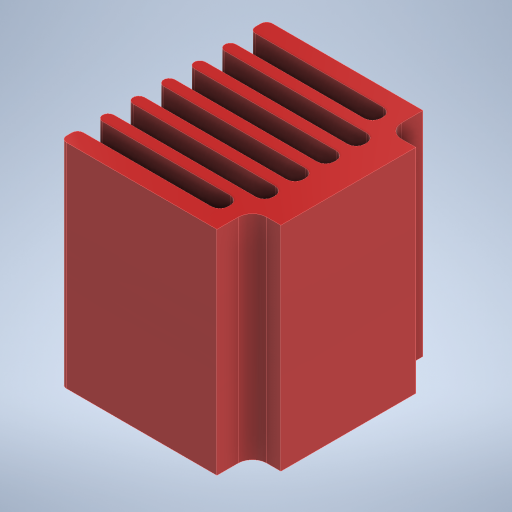
# Autodesk Inventor part: Heatsink5160Pro
Saved by Autodesk Inventor 2023.1 (Build 271208000, 208)
## iProperties
Created: 2022-09-12
Part Number: Heatsink5160Pro
Material: Generisch
Document SubType Name: Modeling
Designer: Rama
Density: 1 g/cm^3
Appearance: Rot
Author: Rama
Autodesk Inventor part; units mm, degrees
ref_plane "YZ Plane" through (0, 0, 0) normal (1, 0, 0) x (0, 1, 0)
ref_plane "XZ Plane" through (0, 0, 0) normal (0, 1, 0) x (-1, 0, 0)
ref_plane "XY Plane" through (0, 0, 0) normal (0, 0, 1) x (1, 0, 0)
sketch "Skizze1" plane through (0, 0, 0) normal (0, 1, 0) x (-1, 0, 0)
  line L0 (6.5, 7.25) -> (-6.5, 7.25)
  line L1 (-6.5, 7.25) -> (-6.5, -7.25)
  line L2 (-6.5, -7.25) -> (6.5, -7.25)
  line L3 (6.5, -7.25) -> (6.5, 7.25)
  line L4 (6.5, 7.25) -> (-6.5, -7.25) construction
  line L5 (-6.5, 7.25) -> (6.5, -7.25) construction
  line L6 (-6.5, -7.25) -> (-4.5, -7.25)
  line L7 (-4.5, -7.25) -> (-4.5, -5.75)
  line L8 (-5.5, -4.75) -> (-6.5, -4.75)
  line L9 (-6.5, -4.75) -> (-6.5, -7.25)
  arc A0 (-4.5, -5.75) -> (-5.5, -4.75) centre (-5.5, -5.75) ccw
  line L10 (-6.5, 0) -> (-5.3357, 0)
  line L11 (6.5, -4.7) -> (-2.9, -4.7)
  line L12 (-3.5, -5.3) -> (-3.5, -5.45)
  line L13 (-2.9, -6.05) -> (6.5, -6.05)
  line L14 (6.5, -6.05) -> (6.5, -4.7)
  line L15 (6.5, -2.55) -> (-3.9, -2.55)
  line L16 (-4.5, -3.15) -> (-4.5, -3.3)
  line L17 (-3.9, -3.9) -> (6.5, -3.9)
  line L18 (6.5, -3.9) -> (6.5, -2.55)
  line L19 (6.5, -0.4) -> (-3.9, -0.4)
  line L20 (-4.5, -1) -> (-4.5, -1.15)
  line L21 (-3.9, -1.75) -> (6.5, -1.75)
  line L22 (6.5, -1.75) -> (6.5, -0.4)
  line L23 (-4.5, 7.25) -> (-4.5, 5.75)
  line L24 (-5.5, 4.75) -> (-6.5, 4.75)
  arc A1 (-5.5, 4.75) -> (-4.5, 5.75) centre (-5.5, 5.75) ccw
  line L25 (6.5, 4.7) -> (-2.9, 4.7)
  line L26 (-3.5, 5.3) -> (-3.5, 5.45)
  line L27 (-2.9, 6.05) -> (6.5, 6.05)
  line L28 (6.5, 2.55) -> (-3.9, 2.55)
  line L29 (-4.5, 3.15) -> (-4.5, 3.3)
  line L30 (-3.9, 3.9) -> (6.5, 3.9)
  line L31 (6.5, 0.4) -> (-3.9, 0.4)
  line L32 (-4.5, 1) -> (-4.5, 1.15)
  line L33 (-3.9, 1.75) -> (6.5, 1.75)
  arc A2 (-2.9, 6.05) -> (-3.5, 5.45) centre (-2.9, 5.45) ccw
  arc A3 (-3.5, 5.3) -> (-2.9, 4.7) centre (-2.9, 5.3) ccw
  arc A4 (-3.9, 3.9) -> (-4.5, 3.3) centre (-3.9, 3.3) ccw
  arc A5 (-4.5, 3.15) -> (-3.9, 2.55) centre (-3.9, 3.15) ccw
  arc A6 (-3.9, 1.75) -> (-4.5, 1.15) centre (-3.9, 1.15) ccw
  arc A7 (-4.5, 1) -> (-3.9, 0.4) centre (-3.9, 1) ccw
  arc A8 (-3.9, -0.4) -> (-4.5, -1) centre (-3.9, -1) ccw
  arc A9 (-4.5, -1.15) -> (-3.9, -1.75) centre (-3.9, -1.15) ccw
  arc A10 (-3.9, -2.55) -> (-4.5, -3.15) centre (-3.9, -3.15) ccw
  arc A11 (-4.5, -3.3) -> (-3.9, -3.9) centre (-3.9, -3.3) ccw
  arc A12 (-2.9, -4.7) -> (-3.5, -5.3) centre (-2.9, -5.3) ccw
  arc A13 (-3.5, -5.45) -> (-2.9, -6.05) centre (-2.9, -5.45) ccw
  point P0 (0, 0)
  point P1 (-4.5, -4.75)
  point P2 (-3.5, -6.05)
  point P3 (-3.5, -4.7)
  point P4 (-4.5, -3.9)
  point P5 (-4.5, -2.55)
  point P6 (-4.5, -1.75)
  point P7 (-4.5, -0.4)
  point P8 (-3.5, 6.05)
  point P9 (-3.5, 4.7)
  point P10 (-4.5, 3.9)
  point P11 (-4.5, 2.55)
  point P12 (-4.5, 1.75)
  point P13 (-4.5, 0.4)
  point P14 (6.5, -3.9)
  point P15 (6.5, -1.75)
  point P16 (6.5, 1.75)
  dimension "d0" = 13
  dimension "d1" = 14.5
  dimension "d2" = 2
  dimension "d3" = 2.5
  dimension "d4" = 1
  dimension "d5" = 10
  dimension "d6" = 1.35
  dimension "d7" = 11
  dimension "d8" = 1.35
  dimension "d9" = 1.2
  dimension "d10" = 0.8
  dimension "d11" = 11
  dimension "d12" = 1.35
  dimension "d13" = 0.8
  dimension "d14" = 0.8
  dimension "d15" = 0.6
  constraints: 68 end point, 29 point on line, 28 point on circle, 26 tangent, 17 symmetric about line, 14 centre point, 11 equal radius, 10 parallel, 6 horizontal, 5 perpendicular, 3 midpoint, 1 other
  measures "d0" distance of L2.end L1.end
  measures "d1" distance of L1.end L0.end
  measures "d2" distance of L8.end point (-4.5, -4.75)
  measures "d3" distance of point (-4.5, -4.75) L6.end
  measures "d4" radius of A0
  measures "d5" distance of L13.end point (-3.5, -6.05)
  measures "d6" distance of point (-3.5, -6.05) point (-3.5, -4.7)
  measures "d7" distance of L17.end point (-4.5, -3.9)
  measures "d8" distance of point (-4.5, -3.9) point (-4.5, -2.55)
  measures "d9" distance between parallel lines of L2 L13
  measures "d10" distance between parallel lines of L17 L11
  measures "d11" distance of L21.end point (-4.5, -1.75)
  measures "d12" distance of point (-4.5, -1.75) point (-4.5, -0.4)
  measures "d13" distance between parallel lines of L15 L21
  measures "d14" distance between parallel lines of L31 L19
  measures "d15" radius of A2
extrude "Extrusion1" add sketch "Skizze1" along normal blind 15 contours L3 L27 A2 L26 A3 L25 L30 A4 L29 A5 L28 L33 A6 L32 A7 L31 L19 A8 L20 A9 L21 L15 A10 L16 A11 L17 L11 A12 L12 A13 L13 L2 L7 A0 L8 L1 L24 A1 L23 L0
fillet "Rundung1" radius 0.4 14 edges at (-6.5, 7.5, 4.7) (-6.5, 7.5, 3.9) (-6.5, 7.5, 2.55) (-6.5, 7.5, 1.75) (-6.5, 7.5, 0.4) (-6.5, 7.5, -0.4) (-6.5, 7.5, -1.75) (-6.5, 7.5, -2.55) (-6.5, 7.5, -3.9) (-6.5, 7.5, -4.7) (-6.5, 7.5, 7.25) (-6.5, 7.5, 6.05) (-6.5, 7.5, -6.05) (-6.5, 7.5, -7.25)
equation "\"d6\" = d8"
equation "\"d13\" = d10"
